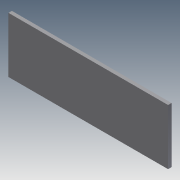
# Autodesk Inventor part: kinect rotate2 bottom
Saved by Autodesk Inventor 2011 (Build 150239000, 239)
## iProperties
Created: 2012-01-14
Part Number: kinect rotate2 bottom
Document SubType Name: Modeling
Designer: Matthew
Density: 1 g/cm^3
Author: Matthew
Autodesk Inventor part; units mm, degrees
ref_plane "YZ Plane" through (0, 0, 0) normal (1, 0, 0) x (0, 1, 0)
ref_plane "XZ Plane" through (0, 0, 0) normal (0, 1, 0) x (-1, 0, 0)
ref_plane "XY Plane" through (0, 0, 0) normal (0, 0, 1) x (1, 0, 0)
sketch "Sketch1" plane through (0, 0, 0) normal (0, 0, 1) x (1, 0, 0)
  line L0 (-39.9518, 9.6865) -> (252.1482, 9.6865)
  line L1 (252.1482, 9.6865) -> (252.1482, -91.9135)
  line L2 (252.1482, -91.9135) -> (-39.9518, -91.9135)
  line L3 (-39.9518, -91.9135) -> (-39.9518, 9.6865)
  point P0 (0, 0)
  dimension "d0" = 292.1
  dimension "d1" = 101.6
  constraints: 8 end point, 2 parallel, 1 horizontal, 1 perpendicular
  measures "d0" distance of L1.end L2.end
  measures "d1" distance of L0.end L1.end
extrude "Extrusion1" add sketch "Sketch1" along normal blind 6.35
sketch "Sketch2" plane through (0, 0, 0) normal (0, 0, -1) x (-1, 0, 0)
  line L0 (39.9518, -91.9135) -> (33.6018, -91.9135)
  line L1 (33.6018, -91.9135) -> (33.6018, -76.6735)
  line L2 (33.6018, -76.6735) -> (39.9518, -76.6735)
  line L3 (39.9518, -76.6735) -> (39.9518, -91.9135)
  line L4 (-252.1482, 9.6865) -> (-245.7982, 9.6865)
  line L5 (-245.7982, 9.6865) -> (-245.7982, -5.5535)
  line L6 (-245.7982, -5.5535) -> (-252.1482, -5.5535)
  line L7 (-252.1482, -5.5535) -> (-252.1482, 9.6865)
  line L8 (-252.1482, -91.9135) -> (-245.7982, -91.9135)
  line L9 (-245.7982, -91.9135) -> (-245.7982, -76.6735)
  line L10 (-245.7982, -76.6735) -> (-252.1482, -76.6735)
  line L11 (-252.1482, -76.6735) -> (-252.1482, -91.9135)
  line L12 (39.9518, 9.6865) -> (33.6018, 9.6865)
  line L13 (33.6018, 9.6865) -> (33.6018, -5.5535)
  line L14 (33.6018, -5.5535) -> (39.9518, -5.5535)
  line L15 (39.9518, -5.5535) -> (39.9518, 9.6865)
  point P0 (0, 0)
  dimension "d4" = 6.35
  dimension "d5" = 15.24
  dimension "d6" = 6.35
  dimension "d7" = 15.24
  constraints: 32 end point, 8 parallel, 4 horizontal, 4 perpendicular
  measures "d4" distance of L1.end L2.end
  measures "d5" distance of L0.end L1.end
  measures "d6" distance of L5.end L6.end
  measures "d7" distance of L4.end L5.end
extrude "Extrusion2" cut sketch "Sketch2" against normal blind 25.4
sketch "Sketch3" plane through (0, 0, 0) normal (0, 0, -1) x (-1, 0, 0)
  line L0 (-252.1482, -76.6735) -> (-258.4982, -76.6735)
  line L1 (-258.4982, -76.6735) -> (-258.4982, -5.5535)
  line L2 (-258.4982, -5.5535) -> (-252.1482, -5.5535)
  line L3 (-252.1482, -5.5535) -> (-252.1482, -76.6735)
  line L4 (39.9518, -76.6735) -> (46.3018, -76.6735)
  line L5 (46.3018, -76.6735) -> (46.3018, -5.5535)
  line L6 (46.3018, -5.5535) -> (39.9518, -5.5535)
  line L7 (39.9518, -5.5535) -> (39.9518, -76.6735)
  point P0 (0, 0)
  dimension "d10" = 6.35
  dimension "d11" = 6.35
  constraints: 16 end point, 4 parallel, 2 horizontal, 2 perpendicular
  measures "d10" distance of L1.end L2.end
  measures "d11" distance of L6.end L5.end
extrude "Extrusion3" add sketch "Sketch3" against normal blind 6.35
sketch "Sketch4" plane through (0, 0, 0) normal (0, 0, -1) x (-1, 0, 0)
  line L0 (33.6018, 9.6865) -> (-245.7982, 9.6865) projected
  line L1 (-258.4982, -76.6735) -> (-245.7982, -76.6735) projected
  line L2 (-106.0982, 9.6865) -> (-106.0982, -25.2385)
  line L3 (-106.0982, -25.2385) -> (-204.0914, -25.2385)
  line L4 (-204.0914, -25.2385) -> (-7.2414, -25.2385)
  circle A0 centre (-7.2414, -25.2385) radius 2.3812
  circle A1 centre (-204.0914, -25.2385) radius 2.3813
  point P0 (0, 0)
  dimension "d14" = 34.925
  dimension "d15" = 97.9932
  dimension "d16" = 196.85
  dimension "d17" = 4.7625
  constraints: 6 end point, 2 centre point, 2 coincident, 2 perpendicular, 1 collinear, 1 midpoint
  measures "d14" distance of L2.start L2.end
  measures "d15" distance of L2.end L3.end
  measures "d16" distance of L3.end L4.end
  measures "d17" diameter of A0
extrude "Extrusion4" cut sketch "Sketch4" against normal blind 6.35
sketch "Sketch5" plane through (0, 0, 0) normal (0, 0, -1) x (-1, 0, 0)
  line L0 (-245.7982, -76.6735) -> (-245.7982, -91.9135) projected
  line L1 (-245.7982, -91.9135) -> (33.6018, -91.9135) projected
  line L2 (33.6018, -91.9135) -> (33.6018, -76.6735) projected
  line L3 (33.6018, -5.5535) -> (33.6018, 9.6865) projected
  line L4 (33.6018, 9.6865) -> (-245.7982, 9.6865) projected
  line L5 (-245.7982, 9.6865) -> (-245.7982, -5.5535) projected
  line L6 (-258.4982, -76.6735) -> (-245.7982, -76.6735) projected
  line L7 (33.6018, -5.5535) -> (-245.7982, -5.5535)
  line L8 (-245.7982, -76.6735) -> (33.6018, -76.6735)
  point P0 (0, 0)
  constraints: 4 end point, 2 parallel
extrude "Extrusion5" cut sketch "Sketch5" against normal blind 6.35
body "Solid1"
